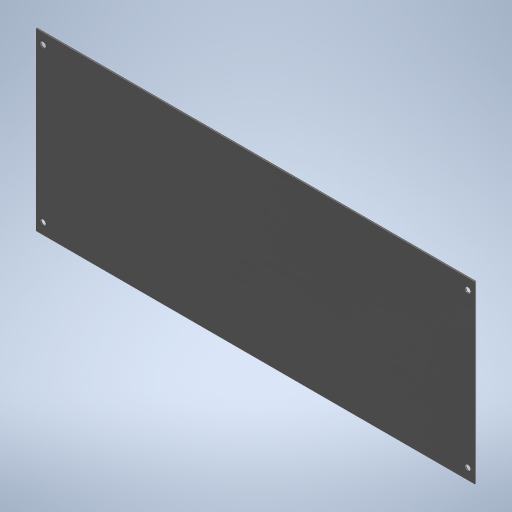
# Autodesk Inventor part: HCMUTE-CDT23-MAT_TRUOT
Saved by Autodesk Inventor 2023 (Build 270158000, 158)
## iProperties
Created: 2023-10-31
Part Number: HCMUTE-CDT23-MAT_TRUOT
Material: PMMA Plastic
Document SubType Name: Sheet Metal
Designer: havie
Density: 1.188 g/cm^3
Sheet Metal Rule: Default_mm
Appearance: Dark Gray
Mass: 256.334 g
Surface Area: 2903.44 cm^2
Volume: 215.769 cm^3
Author: havie
Autodesk Inventor part; units mm, degrees
ref_plane "YZ Plane" through (0, 0, 0) normal (1, 0, 0) x (0, 1, 0)
ref_plane "XZ Plane" through (0, 0, 0) normal (0, 1, 0) x (-1, 0, 0)
ref_plane "XY Plane" through (0, 0, 0) normal (0, 0, 1) x (1, 0, 0)
sketch "Sketch1" plane through (0, 0, 0) normal (0, 0, 1) x (1, 0, 0)
  line L0 (-300, 120) -> (300, 120)
  line L1 (300, 120) -> (300, -120)
  line L2 (300, -120) -> (-300, -120)
  line L3 (-300, -120) -> (-300, 120)
  line L4 (-300, 120) -> (300, -120) construction
  line L5 (300, 120) -> (-300, -120) construction
  point P0 (0, 0)
  dimension "d0" = 600
  dimension "d1" = 240
  measures "d0" distance of L1.end L2.end
  measures "d1" distance of L0.end L1.end
extrude "Plate1" add sketch "Sketch1" along normal mid plane 1.5
sketch "Sketch2" plane through (0, 0, 0.75) normal (0, 0, 1) x (1, 0, 0)
  line L0 (-300, 120) -> (300, 120) projected
  line L1 (-300, -120) -> (-300, 120) projected
  line L2 (300, 120) -> (300, -120) projected
  line L3 (300, -120) -> (-300, -120) projected
  point P0 (0, 0)
  point P1 (-290, 105)
  point P2 (290, 105)
  point P3 (290, -105)
  point P4 (-290, -105)
  dimension "d3" = 15
  dimension "d4" = 10
  dimension "d5" = 10
  dimension "d6" = 15
  constraints: 2 horizontal alignment, 2 vertical alignment
  measures "d3" distance from line of L0 point (-290, 105)
  measures "d4" distance from line of L1 point (-290, 105)
  measures "d5" distance from line of L2 point (290, 105)
  measures "d6" distance from line of L3 point (-290, -105)
hole "Hole1" at (-290, 105, 0.75) at (290, 105, 0.75) at (290, -105, 0.75) at (-290, -105, 0.75) direction (0, 0, -1) diameter 7 end through all
equation "\"d12\" = Thickness"
equation "\"d2\" = Thickness"
equation "\"BendRadius\" = Thickness"
equation "\"BendReliefWidth\" = Thickness"
equation "\"BendReliefDepth\" = 0.5 * Thickness"
equation "\"CornerReliefSize\" = 4 * Thickness"
equation "\"MinimumRemnant\" = 2 * Thickness"
equation "\"TransitionRadius\" = BendRadius"
equation "\"JacobiRadiusSize\" = BendRadius"
equation "\"GapSize\" = Thickness"
equation "\"Thickness\" = 1.5"
body "Solid1"
